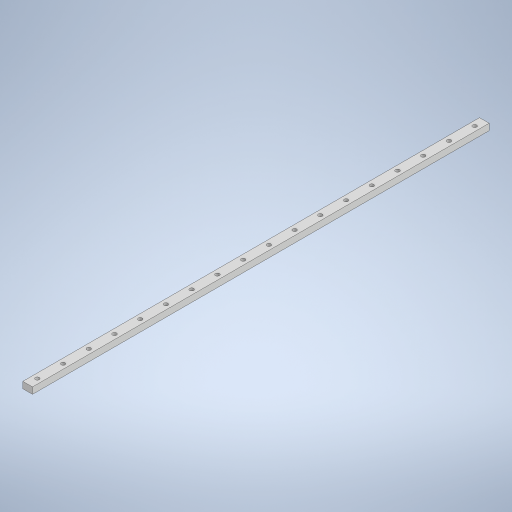
# Autodesk Inventor part: MGN15H-750
Saved by Autodesk Inventor 2023 (Build 270158000, 158)
## iProperties
Created: 2022-04-29
Part Number: MGN15H-750
Material: Generic
Document SubType Name: Modeling
Designer: plebbb
Density: 1 g/cm^3
Appearance: Default
Author: plebbb
Autodesk Inventor part; units mm, degrees
ref_plane "YZ Plane" through (0, 0, 0) normal (1, 0, 0) x (0, 1, 0)
ref_plane "XZ Plane" through (0, 0, 0) normal (0, 1, 0) x (-1, 0, 0)
sketch "Sketch1" plane through (0, 0, 0) normal (0, 0, 1) x (1, 0, 0)
  line L0 (0, 0) -> (15, 0)
  line L1 (15, 0) -> (15, 10)
  line L2 (15, 10) -> (0, 10)
  line L3 (0, 10) -> (0, 0)
  dimension "d0" = 15
  dimension "d1" = 10
  constraints: 9 end point, 2 parallel, 1 horizontal, 1 perpendicular
  measures "d0" distance of L0.start L0.end
  measures "d1" distance of L0.end L1.end
extrude "Extrusion1" add sketch "Sketch1" along normal blind 710
ref_plane "Work Plane1" through (7.5, 10, 710) normal (1, 0, 0) x (0, 0, -1)
sketch "Sketch4" plane through (7.5, 10, 710) normal (1, 0, 0) x (0, 0, -1)
  line L0 (692, 0) -> (692, -4.5)
  line L1 (698, -4.5) -> (698, 0)
  line L2 (692, -4.5) -> (693.25, -4.5)
  line L3 (693.25, -4.5) -> (693.25, -10)
  line L4 (693.25, -10) -> (696.75, -10)
  line L5 (696.75, -10) -> (696.75, -4.5)
  line L6 (696.75, -4.5) -> (698, -4.5)
  line L7 (710, 0) -> (0, 0) projected
  line L8 (710, -10) -> (0, -10) projected
  line L9 (692, 0) -> (698, 0)
  line L10 (695, -10) -> (695, 0)
  point P0 (698, -2.25)
  point P1 (695, 0)
  dimension "d6" = 6
  dimension "d7" = 3.5
  dimension "d8" = 4.5
  dimension "d9" = 15
  constraints: 18 end point, 4 perpendicular, 4 point on line, 3 midpoint, 2 collinear, 2 vertical, 1 horizontal
  measures "d6" distance from line of point (698, -2.25) L0
  measures "d7" distance of L3.end L4.end
  measures "d8" distance of L1.start L1.end
  measures "d9" distance of L8.start L10.start
revolve "Revolution1" cut sketch "Sketch4" angle 360 about axis through (7.5, 0, 15) along (0, -1, 0) contours L7 L1 L6 L5 L4 L10
pattern_linear "Rectangular Pattern1" count 20 spacing 40 along (0, 0, 1) of "Revolution1"
body "Solid1"
